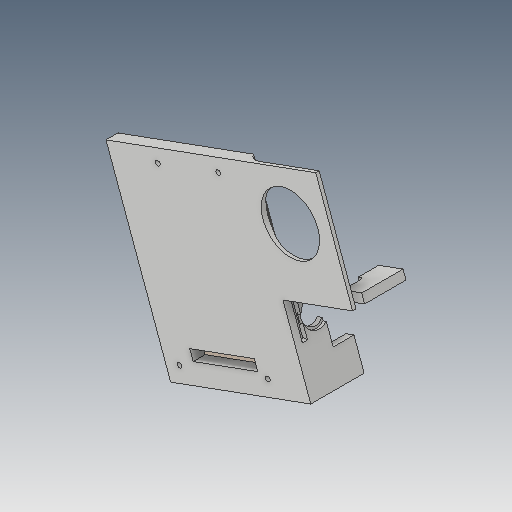
# Autodesk Inventor part: 10_Lidplate_Minispim
Saved by Autodesk Inventor 2019 (Build 230136000, 136)
## iProperties
Created: 2019-08-20
Part Number: 10_Lidplate_Minispim
Material: Generic
Document SubType Name: Modeling
Designer: diederichbenedict
Density: 1 g/cm^3
Appearance: Default
Author: diederichbenedict
Autodesk Inventor part; units mm, degrees
ref_plane "YZ Plane" through (0, 0, 0) normal (1, 0, 0) x (0, 1, 0)
ref_plane "Work Plane1" through (20.4463, 13.7886, 0) normal (0, 0, 1) x (0.9396049, 0.3422611, 0)
sketch "Sketch1" plane through (20.4463, 13.7886, 0) normal (0, 0, 1) x (0.9396049, 0.3422611, 0)
  line L0 (22.1608, -37.7) -> (36, -37.7) projected
  line L1 (-36, -55) -> (-36, -37.7) projected
  line L2 (36, -55) -> (-36, -55) projected
  line L3 (36, -37.7) -> (36, -55) projected
  line L4 (-2, 55) -> (-2, 40.6) projected
  line L5 (-11, 55) -> (-2, 55) projected
  line L6 (-11, 40.6) -> (-11, 55) projected
  line L7 (-2, 40.6) -> (-11, 40.6) projected
  line L8 (36, 55) -> (36, 40.6) projected
  line L9 (25.9, 55) -> (36, 55) projected
  line L10 (25.9, 40.6) -> (25.9, 55) projected
  line L11 (36, 40.6) -> (25.9, 40.6) projected
  line L12 (-36, -37.7) -> (36, -37.7)
  line L13 (36, -37.7) -> (36, 40.6)
  line L14 (36, 40.6) -> (-36, 40.6)
  line L15 (-36, 40.6) -> (-36, -37.7)
  line L16 (-36, 55) -> (36, 55)
  line L17 (36, 55) -> (36, 40.6)
  line L18 (36, 40.6) -> (-36, 40.6)
  line L19 (-36, 40.6) -> (-36, 55)
  circle A0 centre (-6.5, 47.8) radius 1.4 projected
  circle A1 centre (30.95, 47.8) radius 1.4 projected
  circle A2 centre (-27.35, -46.35) radius 1.4 projected
  circle A3 centre (27.35, -46.35) radius 1.4 projected
  line L20 (36, -55) -> (50.8498, -55)
  line L21 (50.8498, -55) -> (50.8498, 55)
  line L22 (50.8498, 55) -> (36, 55)
  line L23 (36, 55) -> (36, -55)
  line L24 (50.8498, 55) -> (94, 55)
  line L25 (94, 55) -> (94, -7.7541)
  line L26 (94, -7.7541) -> (50.8498, -7.7541)
  line L27 (50.8498, -7.7541) -> (50.8498, 55)
  line L28 (94, -55) -> (94, 6.9) construction
  line L29 (-17.8914, -43.5817) -> (-17.8914, -37.7) projected
  line L30 (-36, -37.7) -> (-17.8914, -37.7) projected
  line L31 (22.1608, -37.7) -> (22.1608, -43.5817) projected
  line L32 (22.1608, -43.5817) -> (-17.8914, -43.5817) projected
  point P0 (-23.9307, -5.9579)
  constraints: 32 end point, 8 parallel, 4 horizontal, 4 perpendicular, 2 point on line
extrude "Extrusion1" add sketch "Sketch1" along normal blind 7 contours L12 L15 L14 L7 L11 L13 L0 | L0 L3 L2 L1 L12 L29 L32 L31 | L13 L8 L22 L21 L20 L3 | L11 L10 L9 L8 | L14 L4 L16 L10 | L19 L16 L6 L14 | L21 L24 L25 L26 | L7 L6 L5 L4
sketch "Sketch2" plane through (-32.2038, 53.1455, 0) normal (-0.3422611, 0.9396049, 0) x (0.9396049, 0.3422611, 0)
  line L0 (93, 5.5) -> (146.2403, 5.5) construction
  line L1 (93, 15.5) -> (146.2403, 15.5)
  line L2 (146.2403, -4.5) -> (93, -4.5)
  arc A0 (93, 15.5) -> (93, -4.5) centre (93, 5.5) ccw
  arc A1 (146.2403, -4.5) -> (146.2403, 15.5) centre (146.2403, 5.5) ccw
  line L3 (93, -5) -> (146.2403, -5)
  arc A2 (146.2403, -5) -> (146.2403, 16) centre (146.2403, 5.5) ccw
  line L4 (146.2403, 16) -> (93, 16)
  arc A3 (93, 16) -> (93, -5) centre (93, 5.5) ccw
  ellipse E0 centre (77.2487, -9) end of major axis (77.2487, -19) minor radius 9.9961 (67.2526, -9) -> (77.2487, -19) ccw projected
  ellipse E1 centre (77.2487, -5) end of major axis (77.2487, -15) minor radius 9.9961 (77.2487, 5) -> (67.2526, -5) ccw projected
  point P0 (12.0693, 0)
  point P1 (119.6202, 5.5)
  dimension "d2" = 0.5
  constraints: 12 end point, 8 point on circle, 4 centre point, 4 tangent, 2 parallel, 1 horizontal, 1 midpoint, 5 other
  measures "d2" distance between parallel lines of L2 L3
ref_plane "Work Plane2" through (71.13, 3.9, -15.435) normal (0, -1, 0) x (1, 0, 0)
extrude "Extrusion2" cut sketch "Sketch2" against normal up to surface contours L1 A1 L2 A0 | A3 L4 A2 L3 surface through (71.13, 3.9, -15.435) normal (0, -1, 0)
sketch "Sketch3" plane through (20.4463, 13.7886, 7) normal (0, 0, 1) x (0.9396049, 0.3422611, 0)
  arc A0 (71.0692, 12.0621) -> (74.9801, 44.7417) centre (68.7903, 28.9087) ccw projected
  circle A1 centre (68.7903, 28.9087) radius 17
  point P0 (-23.9307, -5.9579)
  constraints: 1 centre point, 1 coincident, 1 concentric
extrude "Extrusion3" cut sketch "Sketch3" against normal blind 3
sketch "Sketch4" plane through (20.4463, 13.7886, 0) normal (0, 0, -1) x (-0.9396049, -0.3422611, 0)
  line L0 (-48.0557, 55) -> (-48.0557, -28.029) projected
  line L1 (-48.0557, -28.029) -> (-50.8498, -29.0468) projected
  line L2 (-50.8498, -55) -> (-50.8498, -29.0468) projected
  line L3 (36, -55) -> (-50.8498, -55) projected
  line L4 (36, 55) -> (36, -55) projected
  line L5 (-48.0557, 55) -> (36, 55) projected
  circle A0 centre (6.5, 47.8) radius 1.4 projected
  circle A1 centre (-30.95, 47.8) radius 1.4 projected
  circle A2 centre (27.35, -46.35) radius 1.4 projected
  circle A3 centre (-27.35, -46.35) radius 1.4 projected
  line L6 (36, -55) -> (-50.8498, -55) projected
  line L7 (-50.8498, -7.7541) -> (-45.8498, -7.7541)
  line L8 (-45.8498, -7.7541) -> (-45.8498, -55)
  line L9 (-45.8498, -55) -> (-50.8498, -55)
  line L10 (-50.8498, -55) -> (-50.8498, -7.7541)
  line L11 (-50.8498, -7.7541) -> (-94, -7.7541) projected
  line L12 (-94, -7.7541) -> (-45.8498, -7.7541)
  line L13 (-45.8498, -7.7541) -> (-45.8498, -2.7541)
  line L14 (-45.8498, -2.7541) -> (-94, -2.7541)
  line L15 (-94, -2.7541) -> (-94, -7.7541)
  point P0 (23.9307, -5.9579)
  dimension "d8" = 5
  constraints: 16 end point, 4 parallel, 2 horizontal, 2 perpendicular, 2 point on line
  measures "d8" distance between parallel lines of L2 L8
extrude "Extrusion4" add sketch "Sketch4" along normal blind 12 contours L14 L13 L7 L0 | L0 L7 L11 L15 L14 | L7 L8 L3 L2 L1 L0 | L0 L1 L10 L7
sketch "Sketch5" plane through (87.0494, -20.4857, 7) normal (0.9396049, 0.3422611, 0) x (0, 0, -1)
  circle A0 centre (14.5, 35.3) radius 6 projected
  circle A1 centre (14.5, 35.3) radius 6.5
  point P0 (7, 49.0421)
  dimension "d11" = 0.5
  constraints: 1 centre point
  measures "d11" radial gap between concentric circles of A0 A1
extrude "Extrusion5" cut sketch "Sketch5" against normal blind 12 contours A0 | A1
sketch "Sketch6" plane through (70.879, 23.9068, 7) normal (0.3422611, -0.9396049, 0) x (0.9396049, 0.3422611, 0)
  circle A0 centre (11.1502, -14.5) radius 6.25
  ellipse E0 centre (-5.9399, 0) end of major axis (-5.9399, 6) minor radius 5.9977 projected
  point P0 (-74.7806, -7)
  constraints: 1 centre point, 1 other
extrude "Extrusion6" cut sketch "Sketch6" against normal blind 12 contours A0
sketch "Sketch7" plane through (75.1929, 3.9, 0) normal (0, 1, 0) x (1, 0, 0)
  circle A0 centre (13.9443, 7.5) radius 9.75
  ellipse E0 centre (-13.2683, -7) end of major axis (-13.2683, -15.75) minor radius 8.3021 projected
  point P0 (-75.1929, 0)
  constraints: 1 centre point, 1 other
extrude "Extrusion7" cut sketch "Sketch7" along normal up to surface contours A0 surface through (64.4696, 26.8935, 0) normal (-0.3422611, 0.9396049, 0)
sketch "Sketch8" plane through (87.0494, -20.4857, 7) normal (0.9396049, 0.3422611, 0) x (0, 0, -1)
  circle A0 centre (14.5, 35.3) radius 7.5 projected
  circle A1 centre (14.5, 35.3) radius 7.75
  point P0 (7, 49.0421)
  dimension "d20" = 0.25
  constraints: 1 centre point
  measures "d20" radial gap between concentric circles of A0 A1
extrude "Extrusion8" cut sketch "Sketch8" against normal blind 2 contours A0 | A1
sketch "Sketch9" plane through (70.879, 23.9068, 7) normal (0.3422611, -0.9396049, 0) x (0.9396049, 0.3422611, 0)
  circle A0 centre (11.1502, -14.5) radius 7.75
  ellipse E0 centre (-6.1636, 0) end of major axis (-6.1636, -7.5) minor radius 7.4971 projected
  point P0 (-74.7806, -7)
  constraints: 1 centre point, 1 other
extrude "Extrusion9" cut sketch "Sketch9" against normal blind 2 contours A0
sketch "Sketch10" plane through (20.4463, 13.7886, -12) normal (0, 0, -1) x (-0.9396049, -0.3422611, 0)
  line L0 (-45.8498, -2.7541) -> (-45.8498, -55) projected
  line L1 (-48.8498, -24.3904) -> (-48.8498, -26.0097) projected
  line L2 (-48.8498, -26.0097) -> (-50.8498, -26.0097) projected
  line L3 (-50.8498, -26.0097) -> (-50.8498, -55) projected
  line L4 (-50.8498, -55) -> (-45.8498, -55) projected
  line L5 (-45.8498, -55) -> (-45.8498, -24.3904) projected
  line L6 (-45.8498, -24.3904) -> (-48.8498, -24.3904) projected
  line L7 (-57.6627, -5.7541) -> (-55.6903, -5.7541) projected
  line L8 (-57.6627, -2.7541) -> (-57.6627, -5.7541) projected
  line L9 (-81.3083, -2.7541) -> (-94, -2.7541) projected
  line L10 (-94, -2.7541) -> (-94, -7.7541) projected
  line L11 (-55.6903, -7.7541) -> (-50.8498, -7.7541) projected
  line L12 (-55.6903, -5.7541) -> (-55.6903, -7.7541) projected
  line L13 (-50.8498, -55) -> (-50.8498, -7.7541) projected
  line L14 (-45.8498, -55) -> (-50.8498, -55)
  line L15 (-50.8498, -55) -> (-50.8498, -37.6437)
  line L16 (-50.8498, -37.6437) -> (-45.8498, -37.6437)
  line L17 (-45.8498, -37.6437) -> (-45.8498, -55)
  line L18 (-94, -7.7541) -> (-94, 55) projected
  line L19 (-81.3083, -2.7541) -> (-94, -2.7541) projected
  line L20 (-94, -7.7541) -> (-78.9427, -7.7541)
  line L21 (-78.9427, -7.7541) -> (-78.9427, -2.7541)
  line L22 (-78.9427, -2.7541) -> (-94, -2.7541)
  line L23 (-94, -2.7541) -> (-94, -7.7541)
  line L24 (-79.487, -7.7541) -> (-81.3083, -2.7541) projected
  line L25 (-94, -7.7541) -> (-79.487, -7.7541) projected
  line L26 (-50.8498, -7.7541) -> (-50.8498, -13.3903) projected
  line L27 (-50.8498, -13.3903) -> (-48.8498, -13.3903) projected
  line L28 (-48.8498, -13.3903) -> (-48.8498, -15.0096) projected
  line L29 (-48.8498, -15.0096) -> (-45.8498, -15.0096) projected
  line L30 (-45.8498, -15.0096) -> (-45.8498, -2.7541) projected
  line L31 (-45.8498, -2.7541) -> (-57.6627, -2.7541) projected
  point P0 (23.9307, -5.9579)
  point P1 (-66.3373, -2.7541)
  point P2 (-94, 13.5778)
  point P3 (-50.8498, -17.3328)
  constraints: 16 end point, 4 parallel, 2 horizontal, 2 perpendicular, 2 point on line
ref_plane "Work Plane3" through (36, -55, -24.1) normal (0, 0, 1) x (1, 0, 0)
extrude "Extrusion10" add sketch "Sketch10" along normal up to surface (12.1 mm away) contours L0 L4 L3 L16 | L24 L20 L10 L9 | L22 L21 L20 L24
sketch "Sketch11" plane through (109.7118, 43.3734, -24.1) normal (0, 0, -1) x (-0.9396049, -0.3422611, 0)
  circle A0 centre (100.5, 50.5541) radius 1.4 projected
  circle A1 centre (121.35, -43.5959) radius 1.4 projected
  circle A2 centre (66.65, -43.5959) radius 1.4 projected
  circle A3 centre (63.05, 50.5541) radius 1.4 projected
  line L0 (50.6972, 32.0588) -> (50.6972, 12.6454) projected
  line L1 (50.6972, 12.6454) -> (47.5, 12.6454) projected
  line L2 (47.5, 12.6454) -> (47.5, 32.0588) projected
  line L3 (47.5, 32.0588) -> (50.6972, 32.0588) projected
  circle A4 centre (10.9357, -2.5) radius 0.95 projected
  circle A5 centre (45.6502, -49.8414) radius 0.95 projected
  circle A6 centre (48.1, 2.2541) radius 0.95 projected
  circle A7 centre (37.8, -43.5959) radius 0.95 projected
  circle A8 centre (21.1, 3.1232) radius 0.95 projected
  circle A9 centre (45.6502, -38.642) radius 0.95 projected
  circle A10 centre (2.1794, -2.5) radius 0.95 projected
  line L4 (0, 57.7541) -> (130, 57.7541) projected
  line L5 (0, -52.2459) -> (0, 57.7541) projected
  line L6 (130, -52.2459) -> (0, -52.2459) projected
  line L7 (130, 57.7541) -> (130, -52.2459) projected
  point P0 (117.9307, -3.2038)
hole "Hole1" at (83.8774, -19.0821, -24.1) at (80.0443, -8.559, -24.1) at (100.2922, 37.2815, -24.1) at (108.5197, 40.2785, -24.1) direction (0, 0, 1) diameter 1.778 depth 8 tip angle 118
body "Solid1"
